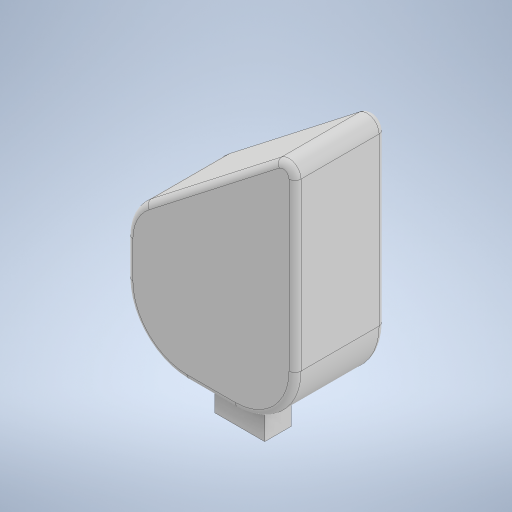
# Autodesk Inventor part: Part3
Saved by Autodesk Inventor 2023.5 (Build 275446020, 446B)
## iProperties
Created: 2025-04-18
Part Number: Part3
Material: Generic
Document SubType Name: Modeling
Designer: Lucky Sah
Density: 1 g/cm^3
Appearance: Default
Author: Lucky Sah
Autodesk Inventor part; units mm, degrees
ref_plane "YZ Plane" through (0, 0, 0) normal (1, 0, 0) x (0, 1, 0)
ref_plane "XZ Plane" through (0, 0, 0) normal (0, 1, 0) x (-1, 0, 0)
ref_plane "XY Plane" through (0, 0, 0) normal (0, 0, 1) x (1, 0, 0)
sketch "Sketch1" plane through (0, 0, 0) normal (0, 0, 1) x (1, 0, 0)
  line L0 (0, 10) -> (0, 16.0873)
  line L1 (10, 0) -> (18, 0)
  line L2 (28, 10) -> (28, 37.6885)
  line L3 (26, 34) -> (18, 34)
  line L4 (24.7721, 39.2672) -> (3.0885, 22.4021)
  arc A0 (18, 0) -> (28, 10) centre (18, 10) ccw
  arc A1 (0, 10) -> (10, 0) centre (10, 10) ccw
  arc A2 (28, 32) -> (26, 34) centre (26, 32) ccw
  arc A3 (28, 37.6885) -> (24.7721, 39.2672) centre (26, 37.6885) ccw
  arc A4 (3.0885, 22.4021) -> (0, 16.0873) centre (8, 16.0873) ccw
  point P0 (0, 0)
  point P1 (0, 20)
  point P2 (28, 0)
  point P3 (28, 34)
  point P4 (2, 0)
  point P5 (0, 2)
  dimension "d0" = 20
  dimension "d1" = 28
  dimension "d2" = 34
  dimension "d3" = 10
  dimension "d18" = 10
  dimension "d19" = 10
  dimension "d21" = 2
  dimension "d22" = 8
  constraints: 14 point on line, 10 end point, 10 point on circle, 10 tangent, 5 centre point, 2 perpendicular, 1 horizontal, 1 vertical
  measures "d0" distance of point (0, 0) point (0, 20)
  measures "d1" distance of point (0, 0) point (28, 0)
  measures "d2" distance of point (28, 0) point (28, 34)
  measures "d3" distance of point (28, 34) L3.end
  measures "d18" radius of A0
  measures "d19" radius of A1
  measures "d21" radius of A3
  measures "d22" radius of A4
extrude "Extrusion1" add sketch "Sketch1" along normal blind 15
fillet "Fillet1" radius 1 5 edges at (25.0711, 2.9289, 15) (14, 0, 15) (0, 13.0437, 15) (28, 23.8442, 15) (13.9303, 30.8347, 15)
fillet "Fillet2" radius 1 5 edges at (28, 23.8442, 0) (25.0711, 2.9289, 0) (14, 0, 0) (0, 13.0437, 0) (13.9303, 30.8347, 0)
sketch "Sketch3" plane through (2, 0, 14) normal (0, -1, 0) x (1, 0, 0)
  line L0 (0, -13) -> (0, 0) projected
  line L1 (24, -14) -> (24, -13) projected
  line L2 (0, 0) -> (24, 0)
  line L3 (24, 0) -> (24, -13)
  line L4 (24, -13) -> (0, -13)
  line L5 (0, -13) -> (0, 0)
  line L6 (9.35, -5.3) -> (14.65, -5.3)
  line L7 (14.65, -5.3) -> (14.65, -6.7)
  line L8 (14.65, -6.7) -> (9.35, -6.7)
  line L9 (9.35, -6.7) -> (9.35, -5.3)
  line L10 (16.15, -3.8) -> (7.85, -3.8)
  line L11 (7.85, -3.8) -> (7.85, -8.2)
  line L12 (7.85, -8.2) -> (16.15, -8.2)
  line L13 (16.15, -8.2) -> (16.15, -3.8)
  point P0 (-2, -14)
  point P1 (12, -6.7)
  point P2 (12, -5.3)
  point P3 (14.65, -6)
  point P4 (9.35, -6)
  dimension "d9" = 1.4
  dimension "d10" = 5.3
  dimension "d11" = 1.5
  dimension "d12" = 24
  dimension "d13" = 9.35
  dimension "d14" = 13
  dimension "d15" = 4.8
  constraints: 24 end point, 6 parallel, 4 midpoint, 3 perpendicular, 2 horizontal, 3 other
  measures "d9" distance of point (12, -6.7) point (12, -5.3)
  measures "d10" distance of point (14.65, -6) point (9.35, -6)
  measures "d11" distance between parallel lines of L6 L10
  measures "d12" distance between parallel lines of L3 L0
  measures "d13" distance between parallel lines of L3 L7
  measures "d14" distance between parallel lines of L4 L2
  measures "d15" distance between parallel lines of L4 L12
extrude "Extrusion2" add sketch "Sketch3" along normal blind 7 contours L13 L12 L11 L10
body "Solid1"
